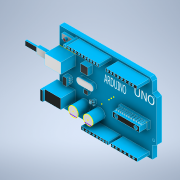
# Autodesk Inventor part: ardUINO
Saved by Autodesk Inventor 2021 (Build 250183000, 183)
## iProperties
Created: 2021-06-25
Part Number: ardUINO
Material: Generic
Document SubType Name: Modeling
Designer: Shaheen Khan
Density: 1 g/cm^3
Appearance: Sky Blue Medium
Author: Shaheen Khan
Autodesk Inventor part; units mm, degrees
ref_plane "YZ Plane" through (0, 0, 0) normal (1, 0, 0) x (0, 1, 0)
ref_plane "XZ Plane" through (0, 0, 0) normal (0, 1, 0) x (-1, 0, 0)
ref_plane "XY Plane" through (0, 0, 0) normal (0, 0, 1) x (1, 0, 0)
sketch "Sketch1" plane through (0, 0, 0) normal (0, 0, 1) x (1, 0, 0)
  line L0 (0, 14.3482) -> (15.8332, 14.3482)
  line L1 (15.8332, 14.3482) -> (15.8332, 9.1942)
  line L2 (15.8332, 9.1942) -> (17.624, 8.3206)
  arc A0 (17.2746, -6.2241) -> (18.0608, -5.831) centre (17.5769, -5.8459) ccw
  line L3 (17.624, 8.3206) -> (17.624, 0)
  line L4 (0, 0) -> (17.624, 0)
  line L5 (0, -14.3482) -> (15.8332, -14.3482)
  line L6 (15.8332, -14.3482) -> (15.8332, -9.1942)
  line L7 (15.8332, -9.1942) -> (17.624, -8.3206)
  line L8 (17.624, -8.3206) -> (17.624, 0)
  line L9 (0, 14.3482) -> (-22.2507, 14.3482)
  line L10 (-22.2507, 14.3482) -> (-22.2507, -14.3482)
  line L11 (-22.2507, -14.3482) -> (0, -14.3482)
  constraints: 24 end point, 4 symmetric about line, 2 horizontal, 2 point on circle, 1 centre point, 1 collinear, 1 vertical
extrude "Extrusion1" add sketch "Sketch1" along normal blind 2
sketch "Sketch2" plane through (0, 0, 2) normal (0, 0, 1) x (1, 0, 0)
  line L0 (-20.2507, 12.9792) -> (-15.9712, 12.9792)
  line L1 (-15.9712, 12.9792) -> (-15.9712, 10.9521)
  line L2 (-15.9712, 10.9521) -> (-20.2507, 10.9521)
  line L3 (-20.2507, 10.9521) -> (-20.2507, 12.9792)
  line L4 (-22.2507, 14.3482) -> (-22.2507, -14.3482) projected
  point P0 (0, 0)
  dimension "d2" = 4.2795
  dimension "d3" = 2
  constraints: 8 end point, 2 parallel, 1 horizontal, 1 perpendicular
  measures "d2" distance of L0.start L0.end
  measures "d3" distance between parallel lines of L4 L3
extrude "Extrusion2" add sketch "Sketch2" along normal blind 1
sketch "Sketch3" plane through (0, 0, 3) normal (0, 0, 1) x (1, 0, 0)
  circle A0 centre (-18.2722, 12.0782) radius 0.6091
  point P0 (0, 0)
  constraints: 1 centre point
extrude "Extrusion3" add sketch "Sketch3" along normal blind 1
sketch "Sketch4" plane through (0, 0, 2) normal (0, 0, 1) x (1, 0, 0)
  circle A0 centre (16.2766, 7.807) radius 0.5
  circle A1 centre (16.2766, -7.9222) radius 0.5
  point P0 (0, 0)
  dimension "d8" = 1
  dimension "d9" = 1
  constraints: 2 centre point
  measures "d8" diameter of A0
  measures "d9" diameter of A1
extrude "Extrusion4" cut sketch "Sketch4" against normal through all contours A0
sketch "Sketch5" plane through (0, 0, 2) normal (0, 0, 1) x (1, 0, 0)
  circle A0 centre (16.2766, -7.2884) radius 0.5
  point P0 (0, 0)
  dimension "d12" = 1
  constraints: 1 centre point
  measures "d12" diameter of A0
extrude "Extrusion5" cut sketch "Sketch5" against normal through all
sketch "Sketch6" plane through (0, 0, 2) normal (0, 0, 1) x (1, 0, 0)
  line L0 (-22.2507, 14.3482) -> (-22.2507, -14.3482) projected
  line L1 (-22.2507, 7.3461) -> (-15.758, 7.3461)
  line L2 (-15.758, 7.3461) -> (-15.758, 3.0825)
  line L3 (-15.758, 3.0825) -> (-22.2507, 3.0825)
  line L4 (-22.2507, 3.0825) -> (-22.2507, 7.3461)
  point P0 (0, 0)
  constraints: 8 end point, 2 parallel, 1 horizontal, 1 perpendicular, 1 point on line
extrude "Extrusion6" add sketch "Sketch6" along normal blind 6
sketch "Sketch7" plane through (0, 0, 2) normal (0, 0, 1) x (1, 0, 0)
  line L0 (-22.2507, 14.3482) -> (-22.2507, -14.3482) projected
  line L1 (-22.2507, -5.3871) -> (-15.758, -5.3871)
  line L2 (-15.758, -5.3871) -> (-15.758, -9.4779)
  line L3 (-15.758, -9.4779) -> (-22.2507, -9.4779)
  line L4 (-22.2507, -9.4779) -> (-22.2507, -5.3871)
  point P0 (0, 0)
  constraints: 8 end point, 2 parallel, 1 horizontal, 1 perpendicular, 1 point on line
extrude "Extrusion7" add sketch "Sketch7" along normal blind 6
sketch "Sketch8" plane through (-22.2507, -14.3482, 0) normal (-1, 0, 0) x (0, 0, 1)
  line L0 (2, 4.8703) -> (8, 4.8703) projected
  line L1 (2, 8.9611) -> (2.5063, 8.9611)
  line L2 (2.5063, 4.8703) -> (2, 4.8703)
  line L3 (2, 8.9611) -> (2, 4.8703) projected
  line L4 (2, 8.9611) -> (8.9017, 8.9611)
  line L5 (8.9017, 8.9611) -> (8.9017, 4.8703)
  line L6 (8.9017, 4.8703) -> (2, 4.8703)
  line L7 (2, 4.8703) -> (2, 8.9611)
  point P0 (0, 14.3482)
  constraints: 12 end point, 3 parallel, 2 horizontal, 1 perpendicular, 1 point on line
extrude "Extrusion8" add sketch "Sketch8" along normal blind 1
sketch "Sketch9" plane through (0, 0, 2) normal (0, 0, 1) x (1, 0, 0)
  point P0 (0, 0)
sketch "Sketch10" plane through (0, 0, 2) normal (0, 0, 1) x (1, 0, 0)
  line L0 (-12.5638, 0) -> (-8.2043, 0) construction
  line L1 (-12.5638, -1.2733) -> (-8.2043, -1.2733)
  line L2 (-8.2043, 1.2733) -> (-12.5638, 1.2733)
  arc A0 (-12.5638, 1.2733) -> (-12.5638, -1.2733) centre (-12.5638, 0) ccw
  arc A1 (-8.2043, -1.2733) -> (-8.2043, 1.2733) centre (-8.2043, 0) ccw
  point P0 (0, 0)
  point P1 (-10.384, 0)
  constraints: 8 end point, 4 point on circle, 4 tangent, 2 centre point, 1 horizontal, 1 midpoint, 1 parallel
extrude "Extrusion9" add sketch "Sketch10" along normal blind 1.5
sketch "Sketch11" plane through (0, 0, 2) normal (0, 0, 1) x (1, 0, 0)
  line L0 (3.026, -3.907) -> (14.8992, -3.907)
  line L1 (14.8992, -3.907) -> (14.8992, -0.8713)
  line L2 (14.8992, -0.8713) -> (3.026, -0.8713)
  line L3 (3.026, -0.8713) -> (3.026, -3.907)
  line L4 (3.026, -3.907) -> (14.8992, -0.8713) construction
  line L5 (14.8992, -3.907) -> (3.026, -0.8713) construction
  point P0 (0, 0)
  point P1 (8.9626, -2.3891)
  constraints: 12 end point, 2 midpoint, 2 parallel, 1 horizontal, 1 perpendicular
extrude "Extrusion10" add sketch "Sketch11" along normal blind 1
sketch "Sketch12" plane through (0, 0, 3) normal (0, 0, 1) x (1, 0, 0)
  line L0 (3.6064, -1.3871) -> (14.4564, -1.3871)
  line L1 (14.4564, -1.3871) -> (14.4564, -3.3598)
  line L2 (14.4564, -3.3598) -> (3.6064, -3.3598)
  line L3 (3.6064, -3.3598) -> (3.6064, -1.3871)
  line L4 (3.6064, -1.3871) -> (14.4564, -3.3598) construction
  line L5 (14.4564, -1.3871) -> (3.6064, -3.3598) construction
  point P0 (0, 0)
  point P1 (9.0314, -2.3734)
  dimension "d25" = 10.85
  constraints: 12 end point, 2 midpoint, 2 parallel, 1 horizontal, 1 perpendicular
  measures "d25" distance of L0.start L0.end
extrude "Extrusion11" add sketch "Sketch12" along normal blind 3
sketch "Sketch13" plane through (0, 0, 2) normal (0, 0, 1) x (1, 0, 0)
  line L0 (15.8332, 9.1942) -> (15.8332, 14.3482) projected
  line L1 (-22.2507, 14.3482) -> (-22.2507, 7.3461) projected
  line L2 (-14.1786, 13.5866) -> (-1.1544, 13.5866)
  line L3 (-1.1544, 13.5866) -> (-1.1544, 12.4026)
  line L4 (-1.1544, 12.4026) -> (-14.1786, 12.4026)
  line L5 (-14.1786, 12.4026) -> (-14.1786, 13.5866)
  line L6 (-13.0538, 13.5866) -> (-13.0538, 12.4026)
  line L7 (-11.3962, 13.5866) -> (-11.3962, 12.4026)
  line L8 (-10.153, 13.5866) -> (-10.153, 12.4026)
  line L9 (-9.0282, 13.5866) -> (-9.0282, 12.4026)
  line L10 (-7.6665, 13.5866) -> (-7.6665, 12.4026)
  line L11 (-6.6601, 13.5866) -> (-6.6601, 12.4026)
  line L12 (-5.0617, 13.5866) -> (-5.0617, 12.4026)
  line L13 (-3.8185, 13.5866) -> (-3.8185, 12.4026)
  line L14 (-2.516, 13.5866) -> (-2.516, 12.4026)
  point P0 (0, 0)
  dimension "d28" = 38.0839
  constraints: 22 end point, 11 vertical, 24 other
  measures "d28" distance between parallel lines of L0 L1
extrude "Extrusion12" add sketch "Sketch13" along normal blind 5
sketch "Sketch14" plane through (0, 0, 7) normal (0, 0, 1) x (1, 0, 0)
  point P0 (0, 0)
sketch "Sketch15" plane through (0, 0, 7) normal (0, 0, 1) x (1, 0, 0)
  circle A0 centre (-13.4005, 13.0295) radius 0.4
  circle A1 centre (-12.0845, 13.0295) radius 0.4
  circle A2 centre (-10.751, 13.0295) radius 0.4
  circle A3 centre (-9.3648, 13.0295) radius 0.4
  circle A4 centre (-8.0664, 13.0295) radius 0.4
  circle A5 centre (-6.6978, 13.0295) radius 0.4
  circle A6 centre (-5.5046, 13.0295) radius 0.4
  circle A7 centre (-4.3115, 13.0295) radius 0.4
  circle A8 centre (-3.1359, 13.0295) radius 0.4
  circle A9 centre (-1.9252, 13.0295) radius 0.4
  point P0 (0, 0)
  dimension "d37" = 0.8
  dimension "d38" = 0.8
  dimension "d39" = 0.8
  dimension "d40" = 0.8
  dimension "d41" = 0.8
  dimension "d42" = 0.8
  dimension "d43" = 0.8
  dimension "d44" = 0.8
  dimension "d45" = 0.8
  dimension "d46" = 0.8
  constraints: 10 centre point
  measures "d37" diameter of A0
  measures "d38" diameter of A1
  measures "d39" diameter of A2
  measures "d40" diameter of A3
  measures "d41" diameter of A4
  measures "d42" diameter of A5
  measures "d43" diameter of A6
  measures "d44" diameter of A7
  measures "d45" diameter of A8
  measures "d46" diameter of A9
extrude "Extrusion13" cut sketch "Sketch15" against normal blind 3
sketch "Sketch16" plane through (0, 0, 2) normal (0, 0, 1) x (1, 0, 0)
  line L0 (1.7477, 13.5866) -> (14.426, 13.5866)
  line L1 (14.426, 13.5866) -> (14.426, 12.4026)
  line L2 (14.426, 12.4026) -> (1.7477, 12.4026)
  line L3 (1.7477, 12.4026) -> (1.7477, 13.5866)
  point P0 (0, 0)
  constraints: 8 end point, 3 perpendicular, 1 horizontal
extrude "Extrusion14" add sketch "Sketch16" along normal blind 5
sketch "Sketch17" plane through (0, 0, 7) normal (0, 0, 1) x (1, 0, 0)
  circle A0 centre (2.4855, 13.0218) radius 0.4
  circle A1 centre (3.8553, 13.0218) radius 0.4
  circle A2 centre (5.1809, 13.0218) radius 0.4
  circle A3 centre (6.6833, 13.0218) radius 0.4
  circle A4 centre (8.1857, 13.0218) radius 0.4
  circle A5 centre (9.7028, 13.0218) radius 0.4
  circle A6 centre (11.3967, 13.0218) radius 0.4
  circle A7 centre (12.8401, 13.0218) radius 0.4
  point P0 (0, 0)
  dimension "d51" = 0.8
  dimension "d52" = 0.8
  dimension "d53" = 0.8
  dimension "d54" = 0.8
  dimension "d55" = 0.8
  dimension "d56" = 0.8
  dimension "d57" = 0.8
  dimension "d58" = 0.8
  constraints: 8 centre point
  measures "d51" diameter of A0
  measures "d52" diameter of A1
  measures "d53" diameter of A2
  measures "d54" diameter of A3
  measures "d55" diameter of A4
  measures "d56" diameter of A5
  measures "d57" diameter of A6
  measures "d58" diameter of A7
extrude "Extrusion15" cut sketch "Sketch17" against normal blind 3
sketch "Sketch18" plane through (0, 0, 2) normal (0, 0, 1) x (1, 0, 0)
  circle A0 centre (-15.1331, 12.9904) radius 0.65
  point P0 (0, 0)
  dimension "d62" = 1.3
  constraints: 1 centre point
  measures "d62" diameter of A0
extrude "Extrusion16" add sketch "Sketch18" along normal blind 5
sketch "Sketch19" plane through (0, 0, 2) normal (0, 0, 1) x (1, 0, 0)
  line L0 (3.7834, -12.1042) -> (14.6065, -12.1042)
  line L1 (14.6065, -12.1042) -> (14.6065, -13.2882)
  line L2 (14.6065, -13.2882) -> (3.7834, -13.2882)
  line L3 (3.7834, -13.2882) -> (3.7834, -12.1042)
  point P0 (0, 0)
  dimension "d65" = 1.184
  constraints: 8 end point, 3 perpendicular, 1 horizontal
  measures "d65" distance of L0.end L1.end
extrude "Extrusion17" add sketch "Sketch19" along normal blind 5
sketch "Sketch20" plane through (0, 0, 7) normal (0, 0, 1) x (1, 0, 0)
  circle A0 centre (4.5665, -12.6575) radius 0.4
  circle A1 centre (6.0338, -12.6575) radius 0.4
  circle A2 centre (7.8143, -12.6575) radius 0.4
  circle A3 centre (9.5288, -12.6575) radius 0.4
  circle A4 centre (11.3196, -12.6575) radius 0.4
  circle A5 centre (13.0566, -12.6575) radius 0.4
  point P0 (0, 0)
  dimension "d68" = 0.8
  dimension "d69" = 0.8
  dimension "d70" = 0.8
  dimension "d71" = 0.8
  dimension "d72" = 0.8
  dimension "d73" = 0.8
  constraints: 6 centre point
  measures "d68" diameter of A0
  measures "d69" diameter of A1
  measures "d70" diameter of A2
  measures "d71" diameter of A3
  measures "d72" diameter of A4
  measures "d73" diameter of A5
extrude "Extrusion18" cut sketch "Sketch20" against normal blind 4
sketch "Sketch21" plane through (-15.1331, 12.9904, 7) normal (0, 0, 1) x (1, 0, 0)
  circle A0 centre (0, 0) radius 0.65 projected
  circle A1 centre (0, 0) radius 0.5
  point P0 (15.1331, -12.9904)
  dimension "d76" = 1
  constraints: 1 centre point, 1 coincident
  measures "d76" diameter of A1
extrude "Extrusion19" cut sketch "Sketch21" against normal through all contours A1
sketch "Sketch22" plane through (0, 0, 2) normal (0, 0, 1) x (1, 0, 0)
  circle A0 centre (-15.4213, -12.2243) radius 0.5
  circle A1 centre (-11.6464, -8.525) radius 2
  circle A2 centre (-5.5689, -8.525) radius 2
  point P0 (0, 0)
  dimension "d79" = 1
  dimension "d80" = 4
  dimension "d81" = 4
  constraints: 3 centre point
  measures "d79" diameter of A0
  measures "d80" diameter of A1
  measures "d81" diameter of A2
extrude "Extrusion20" add sketch "Sketch22" along normal blind 5
sketch "Sketch23" plane through (-15.4213, -12.2243, 7) normal (0, 0, 1) x (1, 0, 0)
  circle A0 centre (0, 0) radius 0.5 projected
  circle A1 centre (0, 0) radius 0.5
  point P0 (15.4213, 12.2243)
  constraints: 1 centre point, 1 coincident
extrude "Extrusion21" cut sketch "Sketch23" against normal through all
sketch "Sketch24" plane through (-11.6464, -8.525, 7) normal (0, 0, 1) x (1, 0, 0)
  circle A0 centre (0, 0) radius 2 projected
  line L0 (-1.4243, -1.404) -> (1.4243, -1.404)
  circle A1 centre (6.0775, 0) radius 2 projected
  line L1 (4.6532, -1.404) -> (7.5018, -1.404)
  point P0 (11.6464, 8.525)
  constraints: 4 end point, 4 point on circle, 2 point on line, 1 horizontal
sketch "Sketch25" plane through (0, 0, 2) normal (0, 0, 1) x (1, 0, 0)
  line L0 (-8.4356, -12.1042) -> (2.6777, -12.1042)
  line L1 (2.6777, -12.1042) -> (2.6777, -13.2882)
  line L2 (2.6777, -13.2882) -> (-8.4356, -13.2882)
  line L3 (-8.4356, -13.2882) -> (-8.4356, -12.1042)
  point P0 (0, 0)
  constraints: 8 end point, 3 perpendicular, 1 horizontal
extrude "Extrusion22" add sketch "Sketch25" along normal blind 5
sketch "Sketch26" plane through (0, 0, 7) normal (0, 0, 1) x (1, 0, 0)
  circle A0 centre (-7.6382, -12.718) radius 0.4
  circle A1 centre (-6.2045, -12.718) radius 0.4
  circle A2 centre (-4.93, -12.718) radius 0.4
  circle A3 centre (-3.3171, -12.718) radius 0.4
  circle A4 centre (-1.8635, -12.718) radius 0.4
  circle A5 centre (-0.4696, -12.718) radius 0.4
  circle A6 centre (0.7053, -12.718) radius 0.4
  circle A7 centre (1.9598, -12.718) radius 0.4
  point P0 (0, 0)
  dimension "d88" = 0.8
  dimension "d89" = 0.8
  dimension "d90" = 0.8
  dimension "d91" = 0.8
  dimension "d92" = 0.8
  dimension "d93" = 0.8
  dimension "d94" = 0.8
  dimension "d95" = 0.8
  constraints: 8 centre point
  measures "d88" diameter of A0
  measures "d89" diameter of A1
  measures "d90" diameter of A2
  measures "d91" diameter of A3
  measures "d92" diameter of A4
  measures "d93" diameter of A5
  measures "d94" diameter of A6
  measures "d95" diameter of A7
extrude "Extrusion23" cut sketch "Sketch26" against normal blind 4
sketch "Sketch27" plane through (0, 0, 2) normal (0, 0, 1) x (1, 0, 0)
  line L0 (-18.9009, -1.0889) -> (-18.9009, -4.0889)
  line L1 (-18.9009, -4.0889) -> (-17.4009, -4.0889)
  line L2 (-17.4009, -4.0889) -> (-17.4009, -1.0889)
  line L3 (-17.4009, -1.0889) -> (-18.9009, -1.0889)
  point P0 (0, 0)
  dimension "d98" = 3
  dimension "d99" = 1.5
  constraints: 8 end point, 3 perpendicular, 1 vertical
  measures "d98" distance of L0.start L0.end
  measures "d99" distance of L0.end L1.end
extrude "Extrusion24" add sketch "Sketch27" along normal blind 2
sketch "Sketch28" plane through (-22.2507, -14.3482, 0) normal (-1, 0, 0) x (0, 0, 1)
  line L0 (6.4079, 20.6615) -> (6.4079, 18.0605)
  line L1 (6.4079, 18.0605) -> (5, 18.0605)
  line L2 (5, 18.0605) -> (5, 20.6615)
  line L3 (5, 20.6615) -> (6.4079, 20.6615)
  point P0 (0, 14.3482)
  constraints: 8 end point, 3 perpendicular, 1 vertical
extrude "Extrusion25" add sketch "Sketch28" along normal blind 5
sketch "Sketch29" plane through (-27.2507, -14.3482, 0) normal (-1, 0, 0) x (0, 0, 1)
  line L0 (5.3675, 20.2831) -> (6.0768, 20.2831)
  line L1 (6.0768, 20.2831) -> (6.0768, 18.4278)
  line L2 (6.0768, 18.4278) -> (5.3675, 18.4278)
  line L3 (5.3675, 18.4278) -> (5.3675, 20.2831)
  point P0 (0, 14.3482)
  constraints: 8 end point, 2 perpendicular, 1 horizontal, 1 vertical
extrude "Extrusion26" add sketch "Sketch29" along normal blind 5
sketch "Sketch30" plane through (0, 0, 2) normal (0, 0, 1) x (1, 0, 0)
  line L0 (-11.6771, 7.0639) -> (-8.6771, 7.0639)
  line L1 (-8.6771, 7.0639) -> (-8.6771, 4.0639)
  line L2 (-8.6771, 4.0639) -> (-11.6771, 4.0639)
  line L3 (-11.6771, 4.0639) -> (-11.6771, 7.0639)
  point P0 (0, 0)
  dimension "d106" = 3
  dimension "d107" = 3
  dimension "d108" = 3
  constraints: 8 end point, 2 perpendicular, 1 horizontal
  measures "d106" distance of L0.start L0.end
  measures "d107" distance of L0.end L1.end
  measures "d108" distance of L1.end L2.end
extrude "Extrusion27" add sketch "Sketch30" along normal blind 2
sketch "Sketch31" plane through (0, 0, 4) normal (0, 0, 1) x (1, 0, 0)
  point P0 (0, 0)
sketch "Sketch32" plane through (0, 0, 2) normal (0, 0, 1) x (1, 0, 0)
  line L0 (-17.4009, -1.0889) -> (-17.4009, -4.0889) projected
  line L1 (-17.4009, -1.3812) -> (-16.7857, -1.3812)
  line L2 (-16.7857, -1.3812) -> (-16.7857, -1.6859)
  line L3 (-16.7857, -1.6859) -> (-17.4009, -1.6859)
  line L4 (-17.4009, -2.1089) -> (-16.7857, -2.1089)
  line L5 (-16.7857, -2.1089) -> (-16.7857, -2.4139)
  line L6 (-16.7857, -2.4139) -> (-17.4009, -2.4139)
  line L7 (-17.4009, -2.9268) -> (-16.7857, -2.9268)
  line L8 (-16.7857, -2.9268) -> (-16.7857, -3.2318)
  line L9 (-16.7857, -3.2318) -> (-17.4009, -3.2318)
  point P0 (0, 0)
  dimension "d111" = 0.3047
  dimension "d112" = 0.305
  dimension "d113" = 0.305
  constraints: 18 end point, 8 point on line, 7 perpendicular, 1 horizontal
  measures "d111" distance of L1.end L2.end
  measures "d112" distance of L4.end L5.end
  measures "d113" distance of L7.end L8.end
extrude "Extrusion28" add sketch "Sketch32" along normal blind 1
sketch "Sketch33" plane through (0, 0, 2) normal (0, 0, 1) x (1, 0, 0)
  line L0 (-18.9009, -4.0889) -> (-18.9009, -1.0889) projected
  line L1 (-18.9009, -1.6593) -> (-19.5455, -1.6593)
  line L2 (-19.5455, -1.6593) -> (-19.5455, -3.52)
  line L3 (-19.5455, -3.52) -> (-18.9009, -3.52)
  point P0 (0, 0)
  constraints: 6 end point, 2 perpendicular, 2 point on line, 1 horizontal
extrude "Extrusion29" add sketch "Sketch33" along normal blind 1
sketch "Sketch34" plane through (0, 0, 2) normal (0, 0, 1) x (1, 0, 0)
  line L0 (-22.2507, 7.3461) -> (-15.758, 7.3461) projected
  arc A0 (-17.7319, 7.3461) -> (-20.7305, 7.3461) centre (-19.2312, 7.122) ccw
  line L1 (-15.758, 3.0825) -> (-22.2507, 3.0825) projected
  arc A1 (-20.7305, 3.0825) -> (-17.7319, 3.0825) centre (-19.2312, 3.7507) ccw
  point P0 (0, 0)
  constraints: 4 point on circle, 4 point on line, 2 centre point
sketch "Sketch35" plane through (0, 0, 2) normal (0, 0, 1) x (1, 0, 0)
  line L0 (-11.7722, -2.3441) -> (-9.7115, -2.3441)
  line L1 (-9.7115, -2.3441) -> (-9.7115, -3.8897)
  line L2 (-9.7115, -3.8897) -> (-11.3086, -3.8897)
  line L3 (-11.3086, -3.8897) -> (-11.3086, -2.3441)
  line L4 (-8.2174, -4.5595) -> (-7.144, -4.5595)
  line L5 (-7.144, -4.5595) -> (-7.144, -6.0344)
  line L6 (-7.144, -6.0344) -> (-7.9321, -6.0344)
  line L7 (-7.9321, -6.0344) -> (-7.9321, -4.5595)
  point P0 (0, 0)
  constraints: 16 end point, 6 perpendicular, 2 horizontal, 2 point on line
extrude "Extrusion30" add sketch "Sketch35" along normal blind 1
sketch "Sketch36" plane through (0, 0, 6) normal (0, 0, 1) x (1, 0, 0)
  circle A0 centre (4.9499, -2.3869) radius 0.75
  circle A1 centre (12.95, -2.3869) radius 0.75
  point P0 (0, 0)
  dimension "d120" = 1.5
  dimension "d121" = 1.5
  constraints: 2 centre point
  measures "d120" diameter of A0
  measures "d121" diameter of A1
extrude "Extrusion31" cut sketch "Sketch36" against normal blind 2
sketch "Sketch37" plane through (0, 0, 3) normal (0, 0, 1) x (1, 0, 0)
  line L0 (14.4564, -1.3871) -> (3.6064, -1.3871) projected
  line L1 (3.842, -1.3871) -> (3.842, -0.8713)
  line L2 (3.026, -0.8713) -> (14.8992, -0.8713) projected
  line L3 (4.2833, -0.8713) -> (4.2833, -1.3871)
  line L4 (4.2833, -1.3871) -> (3.842, -1.3871)
  line L5 (4.7209, -1.3871) -> (4.7209, -0.8713)
  line L6 (5.177, -0.8713) -> (5.177, -1.3871)
  line L7 (4.7209, -0.8713) -> (5.177, -0.8713)
  line L8 (4.7209, -1.3871) -> (5.177, -1.3871)
  line L9 (3.842, -0.8713) -> (4.2833, -0.8713)
  line L10 (3.842, -1.3871) -> (4.2833, -1.3871)
  line L11 (5.6072, -1.3871) -> (5.6072, -0.8713)
  line L12 (5.9929, -0.8713) -> (5.9929, -1.3871)
  line L13 (6.386, -0.8713) -> (6.4119, -1.3871)
  line L14 (6.7929, -0.8713) -> (6.7929, -1.3871)
  line L15 (7.2167, -0.8713) -> (7.2167, -1.3871)
  line L16 (7.6135, -0.8713) -> (7.6135, -1.3871)
  line L17 (8.0585, -0.8713) -> (8.0585, -1.3871)
  line L18 (8.5184, -0.8713) -> (8.5184, -1.3871)
  line L19 (8.9189, -0.8713) -> (8.9189, -1.3871)
  line L20 (9.3747, -0.8713) -> (9.3747, -1.3871)
  line L21 (9.905, -0.8713) -> (9.905, -1.3871)
  line L22 (10.3757, -0.8713) -> (10.3757, -1.3871)
  line L23 (10.9128, -0.8713) -> (10.9128, -1.3871)
  line L24 (11.4417, -0.8713) -> (11.4417, -1.3871)
  line L25 (11.9868, -0.8713) -> (11.9868, -1.3871)
  line L26 (12.4749, -0.8713) -> (12.4749, -1.3871)
  line L27 (13.0051, -0.8713) -> (13.0051, -1.3871)
  line L28 (13.4704, -0.8713) -> (13.4704, -1.3871)
  line L29 (13.8978, -0.8713) -> (13.8978, -1.3871)
  line L30 (14.3361, -0.8713) -> (14.3361, -1.3871)
  line L31 (5.6072, -0.8713) -> (5.9929, -0.8713)
  line L32 (6.386, -0.8713) -> (6.7929, -0.8713)
  line L33 (7.2167, -0.8713) -> (7.6135, -0.8713)
  line L34 (8.0585, -0.8713) -> (8.5184, -0.8713)
  line L35 (8.9189, -0.8713) -> (9.3747, -0.8713)
  line L36 (9.905, -0.8713) -> (10.3757, -0.8713)
  line L37 (10.9128, -0.8713) -> (11.4417, -0.8713)
  line L38 (11.9868, -0.8713) -> (12.4749, -0.8713)
  line L39 (13.0051, -0.8713) -> (13.4704, -0.8713)
  line L40 (13.8978, -0.8713) -> (14.3361, -0.8713)
  point P0 (0, 0)
  constraints: 78 end point, 23 vertical, 14 horizontal, 1 perpendicular, 48 other
sketch "Sketch38" plane through (0, 0, 3) normal (0, 0, 1) x (1, 0, 0)
  line L0 (14.4564, -1.3871) -> (3.6064, -1.3871) projected
  line L1 (5.6232, -1.3871) -> (5.9953, -1.3871)
  line L2 (6.4268, -1.3871) -> (6.8097, -1.3871)
  line L3 (6.8097, -1.3871) -> (7.2304, -1.3871)
  line L4 (7.2304, -1.3871) -> (7.6619, -1.3871)
  line L5 (7.6619, -1.3871) -> (8.0772, -1.4347)
  line L6 (8.0772, -1.4347) -> (8.5194, -1.3871)
  point P0 (0, 0)
  constraints: 12 end point, 7 point on line
extrude "Extrusion32" add sketch "Sketch37" along normal blind 2 contours L0 L29 L2 L30 | L0 L27 L2 L28 | L0 L25 L2 L26 | L0 L23 L2 L24 | L0 L21 L2 L22 | L0 L19 L2 L20 | L0 L17 L2 L18 | L0 L15 L2 L16 | L0 L13 L2 L14 | L0 L11 L2 L12 | L0 L5 L2 L6 | L0 L1 L2 L3
sketch "Sketch39" plane through (0, 0, 3) normal (0, 0, 1) x (1, 0, 0)
  line L0 (14.4564, -3.3598) -> (3.6064, -3.3598) projected
  line L1 (3.8736, -3.3598) -> (3.8736, -3.907)
  line L2 (3.8736, -3.907) -> (4.2884, -3.907)
  line L3 (3.026, -3.907) -> (14.8992, -3.907) projected
  line L4 (4.2884, -3.3598) -> (4.2884, -3.907)
  line L5 (4.737, -3.3598) -> (4.737, -3.907)
  line L6 (4.737, -3.907) -> (5.2872, -3.907)
  line L7 (5.2872, -3.907) -> (5.2872, -3.3598)
  line L8 (5.2872, -3.3598) -> (4.737, -3.3598)
  line L9 (5.6935, -3.3598) -> (5.6935, -3.907)
  line L10 (5.6935, -3.907) -> (6.2353, -3.907)
  line L11 (6.2353, -3.907) -> (6.2353, -3.3598)
  line L12 (6.2353, -3.3598) -> (5.6935, -3.3598)
  line L13 (6.5654, -3.3598) -> (6.5654, -3.907)
  line L14 (6.5654, -3.907) -> (7.0479, -3.907)
  line L15 (7.0479, -3.907) -> (7.0479, -3.3598)
  line L16 (7.0479, -3.3598) -> (6.5654, -3.3598)
  line L17 (7.4373, -3.3598) -> (7.4373, -3.907)
  line L18 (7.4373, -3.907) -> (8.0213, -3.907)
  line L19 (8.0213, -3.907) -> (8.0213, -3.3598)
  line L20 (8.0213, -3.3598) -> (7.4373, -3.3598)
  line L21 (8.4023, -3.3598) -> (8.4023, -3.907)
  line L22 (8.4023, -3.907) -> (8.9271, -3.907)
  line L23 (8.9271, -3.907) -> (8.9271, -3.3598)
  line L24 (8.9271, -3.3598) -> (8.4023, -3.3598)
  line L25 (9.3334, -3.3598) -> (9.3334, -3.907)
  line L26 (9.3334, -3.907) -> (9.909, -3.907)
  line L27 (9.3334, -3.3598) -> (9.909, -3.3598)
  line L28 (10.3915, -3.3598) -> (10.3915, -3.907)
  line L29 (10.9417, -3.3598) -> (10.9417, -3.907)
  line L30 (11.5681, -3.3598) -> (11.5681, -3.9798)
  line L31 (12.1352, -3.3598) -> (12.1352, -3.907)
  line L32 (12.6939, -3.3598) -> (12.6939, -3.907)
  line L33 (13.2271, -3.3598) -> (13.2271, -3.907)
  line L34 (13.8535, -3.3598) -> (13.8535, -3.907)
  line L35 (14.2852, -3.3598) -> (14.2852, -3.907)
  point P0 (0, 0)
  point P1 (11.5681, -3.907)
  constraints: 68 end point, 21 point on line, 16 perpendicular, 9 vertical, 1 parallel, 20 other
extrude "Extrusion33" add sketch "Sketch39" along normal blind 2 contours L34 L3 L33 L0 | L32 L3 L31 L0 | L30 L3 L29 L0 | L28 L3 L25 L0 | L23 L3 L21 L0 | L19 L3 L17 L0 | L15 L3 L13 L0 | L11 L3 L9 L0 | L7 L3 L5 L0 | L4 L2 L1 L0
sketch "Sketch40" plane through (0, 0, 3) normal (0, 0, 1) x (1, 0, 0)
  line L0 (-7.9321, -6.0344) -> (-7.9321, -4.5595) projected
  line L1 (-7.9321, -4.6898) -> (-8.6662, -4.6898)
  line L2 (-8.6662, -4.6898) -> (-8.6662, -5.0068)
  line L3 (-8.6662, -5.0068) -> (-7.9321, -5.0068)
  line L4 (-7.9321, -5.1602) -> (-8.6662, -5.1602)
  line L5 (-8.6662, -5.1602) -> (-8.6662, -5.4567)
  line L6 (-8.6662, -5.4567) -> (-7.9321, -5.4567)
  line L7 (-7.9321, -5.5896) -> (-8.6662, -5.5896)
  line L8 (-8.6662, -5.5896) -> (-8.6662, -5.8963)
  line L9 (-8.6662, -5.8963) -> (-7.9321, -5.8963)
  line L10 (-7.144, -4.5595) -> (-7.144, -6.0344) projected
  line L11 (-7.144, -4.6898) -> (-6.7647, -4.6898)
  line L12 (-6.7647, -4.6898) -> (-6.7647, -4.8957)
  line L13 (-6.7647, -4.8957) -> (-7.144, -4.8957)
  line L14 (-7.144, -5.6445) -> (-6.6919, -5.6445)
  line L15 (-6.6919, -5.6445) -> (-6.6919, -5.9305)
  line L16 (-6.6919, -5.9305) -> (-7.144, -5.8963)
  point P0 (0, 0)
  constraints: 30 end point, 17 point on line, 8 perpendicular, 2 parallel, 1 horizontal
extrude "Extrusion34" add sketch "Sketch40" along normal blind 0.5
chamfer "Chamfer1" distance 1 angle 45 1 edges at (15.8332, 14.3482, 1)
sketch "Sketch41" plane through (0, 0, 2) normal (0, 0, 1) x (1, 0, 0)
  line L0 (-3.9345, 6.3881) -> (5.0894, 6.3881) construction
  line L1 (5.0894, 6.3881) -> (5.0894, 3.2096) construction
  line L2 (5.0894, 3.2096) -> (-3.9345, 3.2096) construction
  line L3 (-3.9345, 3.2096) -> (-3.9345, 6.3881) construction
  line L4 (8.2453, 8.0681) -> (16.7594, 8.0681) construction
  line L5 (16.7594, 8.0681) -> (16.7594, 4.8917) construction
  line L6 (16.7594, 4.8917) -> (8.2453, 4.8917) construction
  line L7 (8.2453, 4.8917) -> (8.2453, 8.0681) construction
  point P0 (0, 0)
  constraints: 4 other
sketch "Sketch42" plane through (0, 0, 2) normal (0, 0, 1) x (1, 0, 0)
  point P0 (0, 0)
body "Solid1"
